# Autodesk Inventor part: Flat Pulley3
Saved by Autodesk Inventor 2014 SP1 (Build 180222100, 222)
## iProperties
Created: 2014-01-12
Part Number: Flat Pulley3
Material: Steel
Document SubType Name: Modeling
Designer: Ryan
Density: 7.85 g/cm^3
Appearance: Steel
CustomPartVersion: 1
Author: Ryan
Autodesk Inventor part; units mm, degrees
ref_plane "YZ Plane" through (0, 0, 0) normal (1, 0, 0) x (0, 1, 0)
ref_plane "XZ Plane" through (0, 0, 0) normal (0, 1, 0) x (-1, 0, 0)
ref_plane "XY Plane" through (0, 0, 0) normal (0, 0, 1) x (1, 0, 0)
sketch "Main Sketch" plane through (0, 0, 0) normal (0, 0, 1) x (1, 0, 0)
  circle A0 centre (0, 0) radius 16.51
  dimension "d0" = 33.02
  constraints: 1 centre point, 1 coincident
  measures "d0" diameter of A0
extrude "Pulley" add sketch "Main Sketch" along normal mid plane 19.111
equation "\"d0\" = da_D"
equation "\"d1\" = da_B"
equation "\"da_D\" = 33.02"
equation "\"da_B\" = 19.11096"
body "Solid1"
